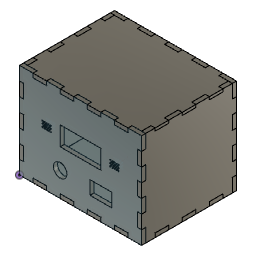
ALARMBOX (Autodesk Fusion 360 design; units mm, degrees)
Autodesk Fusion 360 part; units mm, degrees
note: some values were not read from the file. Set by a fixed rule: which sketch regions a step uses.
(part 1 of 2)
sketch "Sketch1" plane through (0, 0, 0) normal (0, 0, 1) x (1, 0, 0)
sketch "Sketch2" plane through (0, 0, 0) normal (0, 0, 1) x (1, 0, 0)
sketch "Sketch3" plane through (0, 0, 0) normal (0, 1, 0) x (1, 0, 0)
  line L0 (0, 0) -> (90, 0)
  line L1 (90, 0) -> (90, -70)
  line L2 (90, -70) -> (0, -70)
  line L3 (0, -70) -> (0, 0)
  line L4 (0, 0) -> (10, 0)
  line L5 (10, 0) -> (10, -3)
  line L6 (10, -3) -> (20, -3)
  line L7 (20, -3) -> (20, 0)
  line L8 (20, 0) -> (30, 0)
  line L9 (30, 0) -> (30, -3)
  line L10 (30, -3) -> (40, -3)
  line L11 (40, -3) -> (40, 0)
  line L12 (40, 0) -> (50, 0)
  line L13 (50, 0) -> (50, -3)
  line L14 (50, -3) -> (60, -3)
  line L15 (60, -3) -> (60, 0)
  line L16 (60, 0) -> (70, 0)
  line L17 (70, 0) -> (70, -3)
  line L18 (70, -3) -> (80, -3)
  line L19 (80, -3) -> (80, 0)
  line L20 (80, 0) -> (90, 0)
  line L21 (90, 0) -> (90, -3)
  line L22 (90, 0) -> (90, -10)
  line L23 (90, -10) -> (87, -10)
  line L24 (87, -10) -> (87, -20)
  line L25 (87, -20) -> (90, -20)
  line L26 (90, -20) -> (90, -30)
  line L27 (90, -30) -> (87, -30)
  line L28 (87, -30) -> (87, -40)
  line L29 (87, -40) -> (90, -40)
  line L30 (90, -40) -> (90, -50)
  line L31 (90, -50) -> (87, -50)
  line L32 (87, -50) -> (87, -60)
  line L33 (87, -60) -> (90, -60)
  line L34 (90, -60) -> (90, -70)
  line L35 (90, -70) -> (80, -70)
  line L36 (80, -70) -> (80, -67)
  line L37 (80, -67) -> (70, -67)
  line L38 (70, -67) -> (70, -70)
  line L39 (70, -70) -> (60, -70)
  line L40 (60, -70) -> (60, -67)
  line L41 (60, -67) -> (50, -67)
  line L42 (50, -67) -> (50, -70)
  line L43 (50, -70) -> (40, -70)
  line L44 (40, -70) -> (40, -67)
  line L45 (40, -67) -> (30, -67)
  line L46 (30, -67) -> (30, -70)
  line L47 (30, -70) -> (20, -70)
  line L48 (20, -70) -> (20, -67)
  line L49 (20, -67) -> (10, -67)
  line L50 (10, -67) -> (10, -70)
  line L51 (10, -70) -> (0, -70)
  line L52 (0, -70) -> (0, -60)
  line L53 (0, -60) -> (3, -60)
  line L54 (3, -60) -> (3, -50)
  line L55 (3, -50) -> (0, -50)
  line L56 (0, -50) -> (0, -40)
  line L57 (0, -40) -> (3, -40)
  line L58 (3, -40) -> (3, -30)
  line L59 (3, -30) -> (0, -30)
  line L60 (0, -30) -> (0, -20)
  line L61 (0, -20) -> (3, -20)
  line L62 (3, -20) -> (3, -10)
  line L63 (3, -10) -> (0, -10)
  dimension "d7" = 90
  dimension "d8" = 70
  dimension "d9" = 10
  dimension "d14" = 3
  dimension "d15" = 10
  dimension "d16" = 3
  dimension "d17" = 10
  dimension "d18" = 3
  dimension "d19" = 10
  dimension "d20" = 3
  dimension "d21" = 10
  dimension "d22" = 3
  dimension "d23" = 10
  dimension "d24" = 3
  dimension "d25" = 10
  dimension "d26" = 3
  dimension "d27" = 10
  dimension "d28" = 10
  dimension "d29" = 3
  dimension "d30" = 10
  dimension "d31" = 3
  dimension "d32" = 10
  dimension "d33" = 3
  dimension "d34" = 10
  dimension "d35" = 3
  dimension "d36" = 10
  dimension "d37" = 3
  dimension "d38" = 10
  dimension "d39" = 3
  dimension "d40" = 10
  dimension "d41" = 3
  dimension "d42" = 10
  dimension "d43" = 10
  dimension "d44" = 3
  dimension "d45" = 10
  dimension "d46" = 3
  dimension "d47" = 10
  dimension "d48" = 3
  dimension "d49" = 10
  dimension "d50" = 3
  dimension "d51" = 10
  dimension "d52" = 3
  dimension "d53" = 10
  dimension "d54" = 3
  dimension "d55" = 10
  dimension "d56" = 3
  dimension "d57" = 10
  dimension "d58" = 3
  dimension "d59" = 10
  dimension "d60" = 10
  dimension "d61" = 3
  dimension "d62" = 10
  dimension "d63" = 3
  dimension "d64" = 10
  dimension "d65" = 3
  dimension "d66" = 10
  dimension "d67" = 3
  dimension "d68" = 10
  dimension "d69" = 3
  dimension "d70" = 10
  dimension "d71" = 3
  constraint horizontal L0
  constraint vertical L1
  constraint horizontal L2
  constraint vertical L3
  constraint coincident L0.start L3.end
  constraint perpendicular L3 L4
  constraint perpendicular L0 L5
  constraint perpendicular L5 L6
  constraint coincident L0 L7.end
  constraint perpendicular L0 L7
  constraint perpendicular L7 L8
  constraint perpendicular L0 L9
  constraint perpendicular L9 L10
  constraint perpendicular L0 L11
  constraint perpendicular L11 L12
  constraint perpendicular L0 L13
  constraint perpendicular L13 L14
  constraint perpendicular L0 L15
  constraint coincident L0 L16.end
  constraint perpendicular L16 L17
  constraint perpendicular L17 L18
  constraint coincident L0 L19.end
  constraint perpendicular L0 L19
  constraint coincident L0 L1.start
  constraint perpendicular L20 L21
  constraint perpendicular L0 L22
  constraint perpendicular L22 L23
  constraint perpendicular L23 L24
  constraint perpendicular L24 L25
  constraint perpendicular L25 L26
  constraint perpendicular L1 L27
  constraint perpendicular L27 L28
  constraint perpendicular L1 L29
  constraint perpendicular L29 L30
  constraint perpendicular L30 L31
  constraint perpendicular L31 L32
  constraint perpendicular L1 L33
  constraint perpendicular L2 L34
  constraint perpendicular L34 L35
  constraint perpendicular L35 L36
  constraint perpendicular L36 L37
  constraint perpendicular L2 L38
  constraint perpendicular L38 L39
  constraint perpendicular L39 L40
  constraint perpendicular L40 L41
  constraint perpendicular L2 L42
  constraint coincident L2 L43.end
  constraint perpendicular L43 L44
  constraint perpendicular L44 L45
  constraint coincident L2 L46.end
  constraint coincident L2 L47.end
  constraint perpendicular L47 L48
  constraint perpendicular L3 L49
  constraint coincident L2 L50.end
  constraint coincident L2 L3.start
  constraint coincident L3 L52.end
  constraint perpendicular L52 L53
  constraint perpendicular L53 L54
  constraint coincident L3 L55.end
  constraint coincident L3 L56.end
  constraint perpendicular L55 L56
  constraint perpendicular L56 L57
  constraint perpendicular L55 L58
  constraint coincident L3 L59.end
  constraint coincident L3 L60.end
  constraint perpendicular L59 L60
  constraint perpendicular L60 L61
  constraint perpendicular L61 L62
  constraint coincident L3 L63.end
  measures "d7" distance of L0.start L0.end
  measures "d8" distance of L0.start L2.end
  measures "d9" distance of L0.start L4.end
  measures "d14" distance of L4.end L5.end
  measures "d15" distance of L5.end L6.end
  measures "d16" distance of L6.end L7.end
  measures "d17" distance of L7.end L8.end
  measures "d18" distance of L8.end L9.end
  measures "d19" distance of L9.end L10.end
  measures "d20" distance of L10.end L11.end
  measures "d21" distance of L11.end L12.end
  measures "d22" distance of L12.end L13.end
  measures "d23" distance of L13.end L14.end
  measures "d24" distance of L14.end L15.end
  measures "d25" distance of L15.end L16.end
  measures "d26" distance of L16.end L17.end
  measures "d27" distance of L17.end L18.end
  measures "d28" distance of L19.end L0.end
  measures "d29" distance of L0.end L21.end
  measures "d30" distance of L0.end L22.end
  measures "d31" distance of L22.end L23.end
  measures "d32" distance of L23.end L24.end
  measures "d33" distance of L24.end L25.end
  measures "d34" distance of L25.end L26.end
  measures "d35" distance of L26.end L27.end
  measures "d36" distance of L27.end L28.end
  measures "d37" distance of L28.end L29.end
  measures "d38" distance of L29.end L30.end
  measures "d39" distance of L30.end L31.end
  measures "d40" distance of L31.end L32.end
  measures "d41" distance of L32.end L33.end
  measures "d42" distance of L33.end L1.end
  measures "d43" distance of L1.end L35.end
  measures "d44" distance of L35.end L36.end
  measures "d45" distance of L36.end L37.end
  measures "d46" distance of L37.end L38.end
  measures "d47" distance of L38.end L39.end
  measures "d48" distance of L39.end L40.end
  measures "d49" distance of L40.end L41.end
  measures "d50" distance of L41.end L42.end
  measures "d51" distance of L42.end L43.end
  measures "d52" distance of L43.end L44.end
  measures "d53" distance of L44.end L45.end
  measures "d54" distance of L45.end L46.end
  measures "d55" distance of L46.end L47.end
  measures "d56" distance of L47.end L48.end
  measures "d57" distance of L48.end L49.end
  measures "d58" distance of L49.end L50.end
  measures "d59" distance of L50.end L2.end
  measures "d60" distance of L2.end L52.end
  measures "d61" distance of L52.end L53.end
  measures "d62" distance of L53.end L54.end
  measures "d63" distance of L54.end L55.end
  measures "d64" distance of L55.end L56.end
  measures "d65" distance of L56.end L57.end
  measures "d66" distance of L57.end L58.end
  measures "d67" distance of L58.end L59.end
  measures "d68" distance of L59.end L60.end
  measures "d69" distance of L60.end L61.end
  measures "d70" distance of L61.end L62.end
  measures "d71" distance of L62.end L63.end
sketch "Sketch6" plane through (0, 0, 0) normal (0, 0, 1) x (1, 0, 0)
sketch "Sketch7" plane through (0, 0, 0) normal (0, 0, 1) x (1, 0, 0)
  line L0 (0, 0) -> (90, 0)
  line L1 (90, 0) -> (90, 70)
  line L2 (90, 70) -> (0, 70)
  line L3 (0, 70) -> (0, 0)
  dimension "d72" = 90
  dimension "d73" = 70
  constraint horizontal L0
  constraint vertical L1
  constraint horizontal L2
  constraint vertical L3
  constraint coincident L0.start L3.end
  measures "d72" distance of L0.start L0.end
  measures "d73" distance of L0.start L2.end
extrude "Extrude1" add sketch "Sketch7" along normal blind 3 makes body 1
extrude "Extrude2" add sketch "Sketch3" along normal blind 3 separate body contours L0 L1 L2 L3 L4 L5 L6 L7 L8 L9 L10 L11 L12 L13 L14 L15 L16 L17 L18 L19 L20 L21 L22 L23 L24 L25 L26 L27 L28 L29 L30 L31 L32 L33 L34 L35 L36 L37 L38 L39 L40 L41 L42 L43 L44 L45 L46 L47 L48 L49 L50 L51 L52 L53 L54 L55 L56 L57 L58 L59 L60 L61 L62 L63 makes body 2
ref_plane "WorkPlane1" through (45, 35, 1.5) normal (0, 1, 0) x (-1, 0, 0)
mirror "Mirror1" about plane through (45, 35, 1.5) normal (0, 1, 0) of bodies 2 makes body 3
combine "Combine1" operation cut target body 1 tool bodies 2 3 keep tools
sketch "Sketch8" plane through (90, 0, 0) normal (1, 0, 0) x (0, 1, 0)
  line L0 (67, 0) -> (67, 3)
  line L1 (3, 3) -> (3, 0)
  line L2 (3, 0) -> (67, 0)
  line L3 (0, 0) -> (70, 0)
  line L4 (70, 0) -> (70, 70)
  line L5 (70, 70) -> (0, 70)
  line L6 (0, 70) -> (0, 0)
  line L7 (0, 0) -> (10, 0)
  line L8 (10, 0) -> (10.1015, 2.9983)
  line L9 (10.1015, 2.9983) -> (20.1008, 2.8795)
  line L10 (20.1008, 2.8795) -> (20.0677, -0.1203)
  line L11 (20.0677, -0.1203) -> (30.0671, -0.2307)
  line L12 (30.0671, -0.2307) -> (30.0154, 2.7689)
  line L13 (30.0154, 2.7689) -> (40.014, 2.941)
  line L14 (40.014, 2.941) -> (40.0159, -0.059)
  line L15 (40.0159, -0.059) -> (50.0159, -0.0525)
  line L16 (50.0159, -0.0525) -> (50.0001, 2.9475)
  line L17 (50.0001, 2.9475) -> (60, 3)
  line L18 (60, 3) -> (60, 0)
  line L19 (60, 0) -> (70, 0)
  line L20 (60, 70) -> (70, 70)
  line L21 (60, 68) -> (60, 70)
  line L22 (50, 68) -> (60, 68)
  line L23 (50, 70) -> (50, 68)
  line L24 (40, 70) -> (50, 70)
  line L25 (40, 68) -> (40, 70)
  line L26 (30, 68) -> (40, 68)
  line L27 (30, 70) -> (30, 68)
  line L28 (20, 70) -> (30, 70)
  line L29 (20, 68) -> (20, 70)
  line L30 (10, 68) -> (20, 68)
  line L31 (10, 70) -> (10, 68)
  line L32 (0, 70) -> (10, 70)
  dimension "d80" = 70
  dimension "d81" = 70
  dimension "d82" = 10
  dimension "d83" = 3
  dimension "d84" = 10
  dimension "d85" = 3
  dimension "d86" = 10
  dimension "d87" = 3
  dimension "d88" = 10
  dimension "d89" = 3
  dimension "d90" = 10
  dimension "d91" = 3
  dimension "d93" = 10
  dimension "d94" = 3
  constraint horizontal L3
  constraint vertical L4
  constraint horizontal L5
  constraint vertical L6
  constraint coincident L3.start L6.end
  constraint coincident L3 L7.end
  constraint perpendicular L10 L11
  constraint perpendicular L12 L13
  constraint perpendicular L14 L15
  constraint perpendicular L16 L17
  constraint perpendicular L3 L18
  measures "d80" distance of L3.start L3.end
  measures "d81" distance of L3.start L5.end
  measures "d82" distance of L3.start L7.end
  measures "d83" distance of L7.end L8.end
  measures "d84" distance of L8.end L9.end
  measures "d85" distance of L9.end L10.end
  measures "d86" distance of L10.end L11.end
  measures "d87" distance of L11.end L12.end
  measures "d88" distance of L12.end L13.end
  measures "d89" distance of L13.end L14.end
  measures "d90" distance of L14.end L15.end
  measures "d91" distance of L15.end L16.end
  measures "d93" distance of L16.end L17.end
  measures "d94" distance of L17.end L18.end
extrude "Extrude3" add sketch "Sketch8" against normal blind 3 separate body contours L2 L3 L4 L5 L6 L7 L8 L9 L10 L12 L13 L14 L16 L17 L18 L19 L20 L21 L22 L23 L24 L25 L26 L27 L28 L29 L30 L31 L32 makes body 4
ref_plane "WorkPlane2" through (45, 35, 1.5) normal (1, 0, 0) x (0, 1, 0)
mirror "Mirror2" about plane through (45, 35, 1.5) normal (1, 0, 0) of bodies 4 makes body 5
combine "Combine2" operation cut target body 1 tool bodies 4 5 keep tools
combine "Combine3" operation cut target body 4 tool bodies 2 3 keep tools
combine "Combine4" operation cut target body 5 tool bodies 3 2 keep tools
ref_plane "WorkPlane3" through (45, 35, 70) normal (0, 0, -1) x (-1, 0, 0)
sketch "Sketch9" plane through (45, 35, 70) normal (0, 0, -1) x (1, 0, 0)
  line L0 (-45, -35) -> (45, -35)
  line L1 (45, -35) -> (45, 35)
  line L2 (45, 35) -> (-45, 35)
  line L3 (-45, 35) -> (-45, -35)
  dimension "d102" = 90
  dimension "d103" = 70
  constraint horizontal L0
  constraint vertical L1
  constraint horizontal L2
  constraint vertical L3
  measures "d102" distance of L0.start L0.end
  measures "d103" distance of L0.start L2.end
extrude "Extrude4" add sketch "Sketch9" along normal blind 3 separate body makes body 6
combine "Combine5" operation cut target body 6 tool bodies 3 2 5 4 keep tools
sketch "Sketch10" plane through (0, 0, 0) normal (0, -1, 0) x (1, 0, 0)
  line L0 (3, 20) -> (3, 10)
  line L1 (3, 10) -> (0, 10)
  line L2 (0, 10) -> (0, 0)
  line L3 (0, 0) -> (10, 0)
  line L4 (10, 0) -> (10, 3)
  line L5 (10, 3) -> (20, 3)
  line L6 (20, 3) -> (20, 0)
  line L7 (20, 0) -> (30, 0)
  line L8 (30, 0) -> (30, 3)
  line L9 (30, 3) -> (40, 3)
  line L10 (40, 3) -> (40, 0)
  line L11 (40, 0) -> (50, 0)
  line L12 (50, 0) -> (50, 3)
  line L13 (50, 3) -> (60, 3)
  line L14 (60, 3) -> (60, 0)
  line L15 (60, 0) -> (70, 0)
  line L16 (70, 0) -> (70, 3)
  line L17 (70, 3) -> (80, 3)
  line L18 (80, 3) -> (80, 0)
  line L19 (80, 0) -> (90, 0)
  line L20 (90, 0) -> (90, 10)
  line L21 (90, 10) -> (87, 10)
  line L22 (87, 10) -> (87, 20)
  line L23 (87, 20) -> (90, 20)
  line L24 (90, 20) -> (90, 30)
  line L25 (90, 30) -> (87, 30)
  line L26 (87, 30) -> (87, 40)
  line L27 (87, 40) -> (90, 40)
  line L28 (90, 40) -> (90, 50)
  line L29 (90, 50) -> (87, 50)
  line L30 (87, 50) -> (87, 60)
  line L31 (87, 60) -> (90, 60)
  line L32 (90, 60) -> (90, 70)
  line L33 (90, 70) -> (80, 70)
  line L34 (80, 70) -> (80, 67)
  line L35 (80, 67) -> (70, 67)
  line L36 (70, 67) -> (70, 70)
  line L37 (70, 70) -> (60, 70)
  line L38 (60, 70) -> (60, 67)
  line L39 (60, 67) -> (50, 67)
  line L40 (50, 67) -> (50, 70)
  line L41 (50, 70) -> (40, 70)
  line L42 (40, 70) -> (40, 67)
  line L43 (40, 67) -> (30, 67)
  line L44 (30, 67) -> (30, 70)
  line L45 (30, 70) -> (20, 70)
  line L46 (20, 70) -> (20, 67)
  line L47 (20, 67) -> (10, 67)
  line L48 (10, 67) -> (10, 70)
  line L49 (10, 70) -> (0, 70)
  line L50 (0, 70) -> (0, 60)
  line L51 (0, 60) -> (3, 60)
  line L52 (3, 60) -> (3, 50)
  line L53 (3, 50) -> (0, 50)
  line L54 (0, 50) -> (0, 40)
  line L55 (0, 40) -> (3, 40)
  line L56 (3, 40) -> (3, 30)
  line L57 (3, 30) -> (0, 30)
  line L58 (0, 30) -> (0, 20)
  line L59 (0, 20) -> (3, 20)
sketch "Sketch11" plane through (45, 0, 35) normal (0, -1, 0) x (1, 0, 0)
  line L0 (15, 7.25) -> (-15, 7.25)
  line L1 (-15, 7.25) -> (-15, -7.25)
  line L2 (-15, -7.25) -> (15, -7.25)
  line L3 (15, -7.25) -> (15, 7.25)
  line L4 (15, 7.25) -> (-15, -7.25) construction
  line L5 (-15, 7.25) -> (15, -7.25) construction
  dimension "d110" = 30
  dimension "d111" = 14.5
  constraint horizontal L0
  constraint perpendicular L0 L1
  constraint parallel L0 L2
  constraint parallel L1 L3
  constraint coincident L4 origin
  constraint coincident L5 origin
  measures "d110" distance of L1.end L2.end
  measures "d111" distance of L0.end L1.end
sketch "Sketch19" plane through (0, 0, 0) normal (0, -1, 0) x (1, 0, 0)
  line L0 (10, 25) -> (26, 25)
  line L1 (26, 25) -> (26, 15)
  line L2 (26, 15) -> (10, 15)
  line L3 (10, 15) -> (10, 25)
  circle A0 centre (35, 20) radius 5
  circle A1 centre (70, 10) radius 1
  circle A2 centre (75, 10) radius 1
  circle A3 centre (80, 10) radius 1
  circle A4 centre (75, 15) radius 1
  circle A5 centre (80, 15) radius 1
  circle A6 centre (70, 15) radius 1
  circle A7 centre (70, 20) radius 1
  circle A8 centre (75, 20) radius 1
  circle A9 centre (80, 20) radius 1
  dimension "d140" = 16
  dimension "d141" = 2
  constraint horizontal L0
  constraint vertical L1
  constraint horizontal L2
  constraint vertical L3
  measures "d140" distance of L0.start L0.end
  measures "d141" diameter of A1
sketch "Sketch22" plane through (90, 0, 0) normal (1, 0, 0) x (0, 1, 0)
  line L0 (67, 0) -> (67, 10)
  line L1 (67, 10) -> (70, 10)
  line L2 (70, 10) -> (70, 20)
  line L3 (70, 20) -> (67, 20)
  line L4 (67, 20) -> (67, 30)
  line L5 (67, 30) -> (70, 30)
  line L6 (70, 30) -> (70, 40)
  line L7 (70, 40) -> (67, 40)
  line L8 (67, 40) -> (67, 50)
  line L9 (67, 50) -> (70, 50)
  line L10 (70, 50) -> (70, 60)
  line L11 (70, 60) -> (67, 60)
  line L12 (67, 60) -> (67, 70)
  line L13 (67, 70) -> (60, 70)
  line L14 (60, 70) -> (60, 68)
  line L15 (60, 68) -> (50, 68)
  line L16 (50, 68) -> (50, 70)
  line L17 (50, 70) -> (40, 70)
  line L18 (40, 70) -> (40, 68)
  line L19 (40, 68) -> (30, 68)
  line L20 (30, 68) -> (30, 70)
  line L21 (30, 70) -> (20, 70)
  line L22 (20, 70) -> (20, 68)
  line L23 (20, 68) -> (10, 68)
  line L24 (10, 68) -> (10, 70)
  line L25 (10, 70) -> (3, 70)
  line L26 (3, 70) -> (3, 60)
  line L27 (3, 60) -> (0, 60)
  line L28 (0, 60) -> (0, 50)
  line L29 (0, 50) -> (3, 50)
  line L30 (3, 50) -> (3, 40)
  line L31 (3, 40) -> (0, 40)
  line L32 (0, 40) -> (0, 30)
  line L33 (0, 30) -> (3, 30)
  line L34 (3, 30) -> (3, 20)
  line L35 (3, 20) -> (0, 20)
  line L36 (0, 20) -> (0, 10)
  line L37 (0, 10) -> (3, 10)
  line L38 (3, 10) -> (3, 0)
  line L39 (3, 0) -> (10, 0)
  line L40 (10, 0) -> (10.1015, 2.9983)
  line L41 (10.1015, 2.9983) -> (20.1008, 2.8795)
  line L42 (20.1008, 2.8795) -> (20.069, 0)
  line L43 (20.069, 0) -> (30.0631, 0)
  line L44 (30.0631, 0) -> (30.0154, 2.7689)
  line L45 (30.0154, 2.7689) -> (40.014, 2.941)
  line L46 (40.014, 2.941) -> (40.0159, 0)
  line L47 (40.0159, 0) -> (50.0156, 0)
  line L48 (50.0156, 0) -> (50.0001, 2.9475)
  line L49 (50.0001, 2.9475) -> (60, 3)
  line L50 (60, 3) -> (60, 0)
  line L51 (60, 0) -> (67, 0)
  spline S0 degree 3 poles (30.3334, 17.2621) (27.6065, 17.2805) (25.3535, 17.304) (25.3268, 17.3143) knots 0 0 0 0 1 1 1 1
  spline S1 degree 3 poles (25.3268, 17.3143) (25.288, 17.3293) (25.2793, 20.764) (25.2835, 34.3244) knots 0 0 0 0 1 1 1 1
  spline S2 degree 3 poles (25.2835, 34.3244) (25.2865, 43.6695) (25.3034, 52.4586) (25.3211, 53.8556) knots 0 0 0 0 1 1 1 1
  spline S3 degree 3 poles (25.3211, 53.8556) (25.3388, 55.2526) (25.3523, 56.5801) (25.351, 56.8056) knots 0 0 0 0 1 1 1 1
  line L52 (25.351, 56.8056) -> (25.3489, 57.2156)
  line L53 (25.3489, 57.2156) -> (28.7453, 57.2156)
  spline S4 degree 3 poles (28.7453, 57.2156) (30.6133, 57.2156) (34.6484, 57.2036) (37.7122, 57.189) knots 0 0 0 0 1 1 1 1
  line L54 (37.7122, 57.189) -> (43.2827, 57.1624)
  line L55 (43.2827, 57.1624) -> (43.2827, 37.189)
  line L56 (43.2827, 37.189) -> (43.2827, 17.2156)
  line L57 (43.2827, 17.2156) -> (39.2871, 17.2222)
  spline S5 degree 3 poles (39.2871, 17.2222) (37.0895, 17.2258) (33.0604, 17.2438) (30.3335, 17.2621) knots 0 0 0 0 1 1 1 1
  line L58 (30.3335, 17.2621) -> (30.3334, 17.2621)
  spline S6 degree 3 poles (33.2888, 22.5751) (41.3514, 22.6218) (42.7639, 22.6426) (42.7909, 22.7151) knots 0 0 0 0 1 1 1 1
  spline S7 degree 3 poles (42.7909, 22.7151) (42.8012, 22.7428) (42.8305, 24.2032) (42.856, 25.9605) knots 0 0 0 0 1 1 1 1
  line L59 (42.856, 25.9605) -> (42.9023, 29.1556)
  line L60 (42.9023, 29.1556) -> (42.7833, 29.4876)
  spline S8 degree 3 poles (42.7833, 29.4876) (42.5195, 30.2241) (41.9203, 31.2894) (41.3924, 31.9605) knots 0 0 0 0 1 1 1 1
  spline S9 degree 3 poles (41.3924, 31.9605) (40.7567, 32.7688) (39.6052, 33.7374) (38.5579, 34.3448) knots 0 0 0 0 1 1 1 1
  spline S10 degree 3 poles (38.5579, 34.3448) (37.5747, 34.9149) (36.5377, 35.28) (35.5053, 35.4196) knots 0 0 0 0 1 1 1 1
  spline S11 degree 3 poles (35.5053, 35.4196) (34.921, 35.4986) (33.7003, 35.4896) (33.1983, 35.4026) knots 0 0 0 0 1 1 1 1
  spline S12 degree 3 poles (33.1983, 35.4026) (31.3706, 35.086) (29.8426, 34.4023) (28.5057, 33.303) knots 0 0 0 0 1 1 1 1
  spline S13 degree 3 poles (28.5057, 33.303) (27.7205, 32.6573) (27.2357, 32.0549) (26.5364, 30.8556) knots 0 0 0 0 1 1 1 1
  spline S14 degree 3 poles (26.5364, 30.8556) (26.0363, 29.998) (25.8292, 29.5866) (25.7007, 29.1956) knots 0 0 0 0 1 1 1 1
  line L61 (25.7007, 29.1956) -> (25.6087, 28.9156)
  line L62 (25.6087, 28.9156) -> (25.6229, 25.7556)
  spline S15 degree 3 poles (25.6229, 25.7556) (25.6307, 24.0176) (25.6449, 22.5821) (25.6544, 22.5656) knots 0 0 0 0 1 1 1 1
  spline S16 degree 3 poles (25.6544, 22.5656) (25.6758, 22.5283) (25.1001, 22.5276) (33.2888, 22.5751) knots 0 0 0 0 1 1 1 1
  spline S17 degree 3 poles (42.8222, 31.3561) (42.8364, 31.4658) (42.8495, 32.6778) (42.8514, 34.0493) knots 0 0 0 0 1 1 1 1
  line L63 (42.8514, 34.0493) -> (42.8548, 36.5429)
  line L64 (42.8548, 36.5429) -> (42.0114, 37.9893)
  spline S18 degree 3 poles (42.0114, 37.9893) (40.6971, 40.2431) (37.0338, 46.4917) (36.6552, 47.1256) knots 0 0 0 0 1 1 1 1
  spline S19 degree 3 poles (36.6552, 47.1256) (36.468, 47.4391) (36.2989, 47.6956) (36.2795, 47.6956) knots 0 0 0 0 1 1 1 1
  spline S20 degree 3 poles (36.2795, 47.6956) (36.2601, 47.6956) (36.1261, 47.6342) (35.9817, 47.5592) knots 0 0 0 0 1 1 1 1
  spline S21 degree 3 poles (35.9817, 47.5592) (35.8373, 47.4841) (35.6446, 47.4002) (35.5534, 47.3727) knots 0 0 0 0 1 1 1 1
  spline S22 degree 3 poles (35.5534, 47.3727) (35.4623, 47.3452) (35.372, 47.3031) (35.3528, 47.2791) knots 0 0 0 0 1 1 1 1
  spline S23 degree 3 poles (35.3528, 47.2791) (35.331, 47.252) (35.5215, 46.5669) (35.8599, 45.4556) knots 0 0 0 0 1 1 1 1
  spline S24 degree 3 poles (35.8599, 45.4556) (36.4697, 43.4532) (36.8576, 42.1294) (37.8758, 38.5756) knots 0 0 0 0 1 1 1 1
  spline S25 degree 3 poles (37.8758, 38.5756) (38.5788, 36.1222) (38.8741, 35.1608) (39.0062, 34.8956) knots 0 0 0 0 1 1 1 1
  spline S26 degree 3 poles (39.0062, 34.8956) (39.1457, 34.6156) (39.4722, 34.1806) (39.6545, 34.0319) knots 0 0 0 0 1 1 1 1
  spline S27 degree 3 poles (39.6545, 34.0319) (40.6796, 33.1956) (40.9885, 32.8997) (41.487, 32.277) knots 0 0 0 0 1 1 1 1
  spline S28 degree 3 poles (41.487, 32.277) (41.7153, 31.9917) (41.9661, 31.6855) (42.0443, 31.5965) knots 0 0 0 0 1 1 1 1
  spline S29 degree 3 poles (42.0443, 31.5965) (42.2019, 31.4172) (42.647, 31.1277) (42.7381, 31.1453) knots 0 0 0 0 1 1 1 1
  spline S30 degree 3 poles (42.7381, 31.1453) (42.7763, 31.1526) (42.8054, 31.2255) (42.8222, 31.3561) knots 0 0 0 0 1 1 1 1
  spline S31 degree 3 poles (26.0309, 31.2969) (26.3536, 31.4211) (26.5173, 31.5657) (26.921, 32.083) knots 0 0 0 0 1 1 1 1
  spline S32 degree 3 poles (26.921, 32.083) (27.4185, 32.7205) (28.0737, 33.3594) (28.6637, 33.7822) knots 0 0 0 0 1 1 1 1
  spline S33 degree 3 poles (28.6637, 33.7822) (28.9297, 33.9728) (29.1939, 34.1798) (29.2507, 34.2422) knots 0 0 0 0 1 1 1 1
  spline S34 degree 3 poles (29.2507, 34.2422) (29.4833, 34.4975) (29.598, 34.7916) (30.0408, 36.2669) knots 0 0 0 0 1 1 1 1
  spline S35 degree 3 poles (30.0408, 36.2669) (30.2866, 37.0857) (30.909, 39.0426) (31.424, 40.6156) knots 0 0 0 0 1 1 1 1
  spline S36 degree 3 poles (31.424, 40.6156) (31.939, 42.1886) (32.5088, 43.9706) (32.6903, 44.5756) knots 0 0 0 0 1 1 1 1
  spline S37 degree 3 poles (32.6903, 44.5756) (32.8719, 45.1806) (33.1347, 46.0335) (33.2744, 46.4709) knots 0 0 0 0 1 1 1 1
  spline S38 degree 3 poles (33.2744, 46.4709) (33.4853, 47.1311) (33.5196, 47.2751) (33.4766, 47.3182) knots 0 0 0 0 1 1 1 1
  spline S39 degree 3 poles (33.4766, 47.3182) (33.4482, 47.3468) (33.2411, 47.451) (33.0166, 47.5499) knots 0 0 0 0 1 1 1 1
  spline S40 degree 3 poles (33.0166, 47.5499) (32.6354, 47.7177) (32.604, 47.7252) (32.5447, 47.6626) knots 0 0 0 0 1 1 1 1
  spline S41 degree 3 poles (32.5447, 47.6626) (32.5098, 47.6258) (31.9776, 46.7496) (31.3621, 45.7156) knots 0 0 0 0 1 1 1 1
  spline S42 degree 3 poles (31.3621, 45.7156) (29.4896, 42.5702) (27.0499, 38.4924) (26.0731, 36.8756) knots 0 0 0 0 1 1 1 1
  line L65 (26.0731, 36.8756) -> (25.6865, 36.2356)
  line L66 (25.6865, 36.2356) -> (25.6657, 33.7756)
  spline S43 degree 3 poles (25.6657, 33.7756) (25.6542, 32.4226) (25.6517, 31.2931) (25.6601, 31.2656) knots 0 0 0 0 1 1 1 1
  spline S44 degree 3 poles (25.6601, 31.2656) (25.6818, 31.1945) (25.7881, 31.2035) (26.0309, 31.2969) knots 0 0 0 0 1 1 1 1
  spline S45 degree 3 poles (30.8329, 35.052) (31.6951, 35.4257) (32.7366, 35.6956) (33.3163, 35.6956) knots 0 0 0 0 1 1 1 1
  spline S46 degree 3 poles (33.3163, 35.6956) (33.6245, 35.6956) (33.7747, 35.7589) (33.9553, 35.9647) knots 0 0 0 0 1 1 1 1
  line L67 (33.9553, 35.9647) -> (34.0968, 36.1261)
  line L68 (34.0968, 36.1261) -> (34.1203, 36.7009)
  spline S47 degree 3 poles (34.1203, 36.7009) (34.1332, 37.017) (34.1482, 39.5076) (34.1537, 42.2356) knots 0 0 0 0 1 1 1 1
  line L69 (34.1537, 42.2356) -> (34.1637, 47.1956)
  line L70 (34.1637, 47.1956) -> (34.0373, 47.2081)
  spline S48 degree 3 poles (34.0373, 47.2081) (33.9296, 47.2188) (33.9048, 47.2042) (33.8696, 47.109) knots 0 0 0 0 1 1 1 1
  spline S49 degree 3 poles (33.8696, 47.109) (33.8263, 46.9917) (32.6937, 43.3148) (31.9865, 40.9956) knots 0 0 0 0 1 1 1 1
  spline S50 degree 3 poles (31.9865, 40.9956) (31.7584, 40.2476) (31.2669, 38.6538) (30.8943, 37.4539) knots 0 0 0 0 1 1 1 1
  spline S51 degree 3 poles (30.8943, 37.4539) (30.5216, 36.2539) (30.2167, 35.2067) (30.2167, 35.1267) knots 0 0 0 0 1 1 1 1
  spline S52 degree 3 poles (30.2167, 35.1267) (30.2167, 35.0018) (30.2936, 34.8556) (30.3594, 34.8556) knots 0 0 0 0 1 1 1 1
  spline S53 degree 3 poles (30.3594, 34.8556) (30.3706, 34.8556) (30.5837, 34.944) (30.8329, 35.052) knots 0 0 0 0 1 1 1 1
  spline S54 degree 3 poles (38.3815, 34.973) (38.4463, 35.0976) (38.4305, 35.201) (38.268, 35.7146) knots 0 0 0 0 1 1 1 1
  spline S55 degree 3 poles (38.268, 35.7146) (38.1196, 36.1839) (37.7415, 37.5168) (36.3216, 42.5756) knots 0 0 0 0 1 1 1 1
  spline S56 degree 3 poles (36.3216, 42.5756) (35.4602, 45.6445) (35.297, 46.2195) (35.1326, 46.7656) knots 0 0 0 0 1 1 1 1
  line L71 (35.1326, 46.7656) -> (34.9971, 47.2156)
  line L72 (34.9971, 47.2156) -> (34.7457, 47.2156)
  spline S57 degree 3 poles (34.7457, 47.2156) (34.5722, 47.2156) (34.4932, 47.2001) (34.4908, 47.1656) knots 0 0 0 0 1 1 1 1
  spline S58 degree 3 poles (34.4908, 47.1656) (34.4778, 46.9728) (34.4992, 40.6508) (34.5197, 38.639) knots 0 0 0 0 1 1 1 1
  line L73 (34.5197, 38.639) -> (34.545, 36.1624)
  line L74 (34.545, 36.1624) -> (34.6815, 36.0069)
  spline S59 degree 3 poles (34.6815, 36.0069) (34.7566, 35.9214) (34.8546, 35.8313) (34.8992, 35.8066) knots 0 0 0 0 1 1 1 1
  spline S60 degree 3 poles (34.8992, 35.8066) (34.9438, 35.782) (35.2341, 35.7289) (35.5442, 35.6885) knots 0 0 0 0 1 1 1 1
  spline S61 degree 3 poles (35.5442, 35.6885) (36.226, 35.5999) (37.0666, 35.3717) (37.7041, 35.1022) knots 0 0 0 0 1 1 1 1
  spline S62 degree 3 poles (37.7041, 35.1022) (38.2287, 34.8805) (38.3239, 34.8623) (38.3815, 34.973) knots 0 0 0 0 1 1 1 1
  spline S63 degree 3 poles (42.8081, 39.0236) (42.8434, 39.0599) (42.8548, 39.6648) (42.8548, 41.5012) knots 0 0 0 0 1 1 1 1
  line L75 (42.8548, 41.5012) -> (42.8548, 43.9307)
  line L76 (42.8548, 43.9307) -> (42.695, 44.1232)
  spline S64 degree 3 poles (42.695, 44.1232) (42.1455, 44.7851) (41.8818, 45.0114) (40.6383, 45.8881) knots 0 0 0 0 1 1 1 1
  spline S65 degree 3 poles (40.6383, 45.8881) (39.9646, 46.363) (38.9044, 47.1142) (38.2823, 47.5572) knots 0 0 0 0 1 1 1 1
  spline S66 degree 3 poles (38.2823, 47.5572) (37.6601, 48.0003) (37.1291, 48.3769) (37.1021, 48.394) knots 0 0 0 0 1 1 1 1
  spline S67 degree 3 poles (37.1021, 48.394) (37.0494, 48.4276) (36.633, 48.0355) (36.633, 47.9523) knots 0 0 0 0 1 1 1 1
  spline S68 degree 3 poles (36.633, 47.9523) (36.633, 47.9128) (37.6617, 46.1622) (40.3567, 41.6156) knots 0 0 0 0 1 1 1 1
  spline S69 degree 3 poles (40.3567, 41.6156) (41.5801, 39.5517) (41.7611, 39.2653) (41.8959, 39.1796) knots 0 0 0 0 1 1 1 1
  spline S70 degree 3 poles (41.8959, 39.1796) (42.1555, 39.0145) (42.7075, 38.9201) (42.8081, 39.0236) knots 0 0 0 0 1 1 1 1
  spline S71 degree 3 poles (26.7408, 39.194) (27.0325, 39.3422) (27.0391, 39.3491) (27.3172, 39.7898) knots 0 0 0 0 1 1 1 1
  spline S72 degree 3 poles (27.3172, 39.7898) (27.4719, 40.035) (28.4267, 41.6306) (29.439, 43.3356) knots 0 0 0 0 1 1 1 1
  spline S73 degree 3 poles (29.439, 43.3356) (30.4513, 45.0406) (31.4866, 46.7822) (31.7397, 47.2059) knots 0 0 0 0 1 1 1 1
  spline S74 degree 3 poles (31.7397, 47.2059) (31.9928, 47.6295) (32.1999, 47.9902) (32.1999, 48.0074) knots 0 0 0 0 1 1 1 1
  spline S75 degree 3 poles (32.1999, 48.0074) (32.1999, 48.0246) (32.1145, 48.1252) (32.01, 48.231) knots 0 0 0 0 1 1 1 1
  spline S76 degree 3 poles (32.01, 48.231) (31.8348, 48.4085) (31.813, 48.4195) (31.7281, 48.373) knots 0 0 0 0 1 1 1 1
  spline S77 degree 3 poles (31.7281, 48.373) (31.6142, 48.3107) (28.1451, 45.9343) (27.2419, 45.2999) knots 0 0 0 0 1 1 1 1
  spline S78 degree 3 poles (27.2419, 45.2999) (26.5014, 44.7798) (26.1506, 44.4447) (25.8896, 44.0081) knots 0 0 0 0 1 1 1 1
  line L77 (25.8896, 44.0081) -> (25.7147, 43.7156)
  line L78 (25.7147, 43.7156) -> (25.6896, 41.5756)
  spline S79 degree 3 poles (25.6896, 41.5756) (25.6661, 39.5716) (25.6689, 39.4267) (25.7338, 39.2956) knots 0 0 0 0 1 1 1 1
  spline S80 degree 3 poles (25.7338, 39.2956) (25.8911, 38.9779) (26.2455, 38.9421) (26.7408, 39.194) knots 0 0 0 0 1 1 1 1
  line L79 (42.7932, 45.7097) -> (42.8937, 45.7775)
  line L80 (42.8937, 45.7775) -> (42.8937, 47.3319)
  line L81 (42.8937, 47.3319) -> (42.8937, 48.8863)
  line L82 (42.8937, 48.8863) -> (42.7394, 49.0297)
  spline S81 degree 3 poles (42.7394, 49.0297) (42.6545, 49.1086) (42.4926, 49.2352) (42.3797, 49.3111) knots 0 0 0 0 1 1 1 1
  spline S82 degree 3 poles (42.3797, 49.3111) (42.1783, 49.4463) (42.1355, 49.4559) (40.2105, 49.7968) knots 0 0 0 0 1 1 1 1
  spline S83 degree 3 poles (40.2105, 49.7968) (39.1305, 49.9881) (38.1616, 50.1471) (38.0575, 50.1501) knots 0 0 0 0 1 1 1 1
  line L83 (38.0575, 50.1501) -> (37.8683, 50.1556)
  line L84 (37.8683, 50.1556) -> (37.7411, 49.7444)
  spline S84 degree 3 poles (37.7411, 49.7444) (37.6711, 49.5182) (37.5421, 49.2057) (37.4544, 49.0499) knots 0 0 0 0 1 1 1 1
  spline S85 degree 3 poles (37.4544, 49.0499) (37.3667, 48.894) (37.3059, 48.7482) (37.3194, 48.7258) knots 0 0 0 0 1 1 1 1
  spline S86 degree 3 poles (37.3194, 48.7258) (37.34, 48.6916) (40.5958, 46.4588) (41.4284, 45.908) knots 0 0 0 0 1 1 1 1
  spline S87 degree 3 poles (41.4284, 45.908) (41.5743, 45.8115) (41.7843, 45.7064) (41.8951, 45.6744) knots 0 0 0 0 1 1 1 1
  spline S88 degree 3 poles (41.8951, 45.6744) (42.1597, 45.5979) (42.6563, 45.6175) (42.7932, 45.7097) knots 0 0 0 0 1 1 1 1
  spline S89 degree 3 poles (27.2079, 45.8294) (27.3122, 45.8845) (27.9924, 46.3436) (28.7196, 46.8497) knots 0 0 0 0 1 1 1 1
  spline S90 degree 3 poles (28.7196, 46.8497) (29.4468, 47.3557) (30.3439, 47.9797) (30.7132, 48.2362) knots 0 0 0 0 1 1 1 1
  spline S91 degree 3 poles (30.7132, 48.2362) (31.0825, 48.4928) (31.4092, 48.728) (31.4393, 48.7589) knots 0 0 0 0 1 1 1 1
  spline S92 degree 3 poles (31.4393, 48.7589) (31.4862, 48.8071) (31.4639, 48.8758) (31.2817, 49.2453) knots 0 0 0 0 1 1 1 1
  spline S93 degree 3 poles (31.2817, 49.2453) (31.165, 49.482) (31.0414, 49.7971) (31.007, 49.9456) knots 0 0 0 0 1 1 1 1
  spline S94 degree 3 poles (31.007, 49.9456) (30.9518, 50.1836) (30.9336, 50.2156) (30.8535, 50.2156) knots 0 0 0 0 1 1 1 1
  spline S95 degree 3 poles (30.8535, 50.2156) (30.7483, 50.2156) (27.8067, 49.7712) (27.1474, 49.6557) knots 0 0 0 0 1 1 1 1
  spline S96 degree 3 poles (27.1474, 49.6557) (26.5905, 49.5581) (26.3602, 49.4426) (25.9886, 49.0748) knots 0 0 0 0 1 1 1 1
  line L85 (25.9886, 49.0748) -> (25.7049, 48.794)
  line L86 (25.7049, 48.794) -> (25.7151, 47.3948)
  line L87 (25.7151, 47.3948) -> (25.7254, 45.9956)
  line L88 (25.7254, 45.9956) -> (25.9755, 45.8596)
  spline S97 degree 3 poles (25.9755, 45.8596) (26.3809, 45.6391) (26.8272, 45.6282) (27.2079, 45.8294) knots 0 0 0 0 1 1 1 1
  spline S98 degree 3 poles (35.263, 47.5559) (35.7346, 47.6703) (36.1958, 47.9685) (36.6383, 48.4452) knots 0 0 0 0 1 1 1 1
  spline S99 degree 3 poles (36.6383, 48.4452) (37.0899, 48.9319) (37.4148, 49.5054) (37.5505, 50.0554) knots 0 0 0 0 1 1 1 1
  spline S100 degree 3 poles (37.5505, 50.0554) (37.6466, 50.4452) (37.6093, 51.2646) (37.4713, 51.7956) knots 0 0 0 0 1 1 1 1
  spline S101 degree 3 poles (37.4713, 51.7956) (37.3268, 52.3515) (37.1584, 52.6441) (36.7342, 53.0763) knots 0 0 0 0 1 1 1 1
  spline S102 degree 3 poles (36.7342, 53.0763) (36.1201, 53.702) (35.5016, 54.0102) (34.6068, 54.1362) knots 0 0 0 0 1 1 1 1
  spline S103 degree 3 poles (34.6068, 54.1362) (33.7711, 54.2539) (32.7766, 53.824) (32.0447, 53.0287) knots 0 0 0 0 1 1 1 1
  spline S104 degree 3 poles (32.0447, 53.0287) (31.7828, 52.7441) (31.6955, 52.6127) (31.5213, 52.2414) knots 0 0 0 0 1 1 1 1
  spline S105 degree 3 poles (31.5213, 52.2414) (31.4064, 51.9962) (31.2901, 51.6966) (31.263, 51.5756) knots 0 0 0 0 1 1 1 1
  spline S106 degree 3 poles (31.263, 51.5756) (31.1943, 51.2695) (31.2026, 50.4951) (31.278, 50.1756) knots 0 0 0 0 1 1 1 1
  spline S107 degree 3 poles (31.278, 50.1756) (31.6149, 48.7471) (32.6679, 47.7107) (33.9573, 47.5385) knots 0 0 0 0 1 1 1 1
  spline S108 degree 3 poles (33.9573, 47.5385) (34.3672, 47.4838) (35.0004, 47.4922) (35.263, 47.5559) knots 0 0 0 0 1 1 1 1
  spline S109 degree 3 poles (42.3764, 50.1384) (42.5089, 50.1837) (42.6752, 50.2608) (42.7458, 50.3098) knots 0 0 0 0 1 1 1 1
  line L89 (42.7458, 50.3098) -> (42.8742, 50.3988)
  line L90 (42.8742, 50.3988) -> (42.8742, 51.397)
  line L91 (42.8742, 51.397) -> (42.8742, 52.3952)
  line L92 (42.8742, 52.3952) -> (42.6448, 52.4888)
  spline S110 degree 3 poles (42.6448, 52.4888) (42.485, 52.554) (42.2724, 52.5948) (41.9448, 52.6231) knots 0 0 0 0 1 1 1 1
  line L93 (41.9448, 52.6231) -> (41.4743, 52.6636)
  line L94 (41.4743, 52.6636) -> (39.7828, 52.2984)
  spline S111 degree 3 poles (39.7828, 52.2984) (37.5924, 51.8255) (37.7868, 51.8843) (37.8129, 51.703) knots 0 0 0 0 1 1 1 1
  spline S112 degree 3 poles (37.8129, 51.703) (37.8246, 51.6219) (37.8544, 51.3486) (37.8792, 51.0956) knots 0 0 0 0 1 1 1 1
  spline S113 degree 3 poles (37.8792, 51.0956) (37.9039, 50.8426) (37.9309, 50.6283) (37.9392, 50.6194) knots 0 0 0 0 1 1 1 1
  spline S114 degree 3 poles (37.9392, 50.6194) (37.9474, 50.6105) (38.79, 50.4717) (39.8115, 50.311) knots 0 0 0 0 1 1 1 1
  spline S115 degree 3 poles (39.8115, 50.311) (41.8101, 49.9965) (41.9361, 49.988) (42.3764, 50.1384) knots 0 0 0 0 1 1 1 1
  spline S116 degree 3 poles (28.819, 50.3539) (29.9003, 50.496) (30.8134, 50.6234) (30.8481, 50.6371) knots 0 0 0 0 1 1 1 1
  spline S117 degree 3 poles (30.8481, 50.6371) (30.8937, 50.6551) (30.9179, 50.7357) (30.9356, 50.9288) knots 0 0 0 0 1 1 1 1
  spline S118 degree 3 poles (30.9356, 50.9288) (30.949, 51.0755) (30.979, 51.3271) (31.0023, 51.4878) knots 0 0 0 0 1 1 1 1
  spline S119 degree 3 poles (31.0023, 51.4878) (31.028, 51.6648) (31.0307, 51.7944) (31.0091, 51.8166) knots 0 0 0 0 1 1 1 1
  spline S120 degree 3 poles (31.0091, 51.8166) (30.9687, 51.8581) (27.7097, 52.5973) (27.332, 52.6507) knots 0 0 0 0 1 1 1 1
  spline S121 degree 3 poles (27.332, 52.6507) (26.9138, 52.7097) (26.3779, 52.6072) (25.9392, 52.3843) knots 0 0 0 0 1 1 1 1
  line L95 (25.9392, 52.3843) -> (25.7254, 52.2756)
  line L96 (25.7254, 52.2756) -> (25.7148, 51.5257)
  line L97 (25.7148, 51.5257) -> (25.7042, 50.7757)
  line L98 (25.7042, 50.7757) -> (25.8605, 50.6013)
  spline S122 degree 3 poles (25.8605, 50.6013) (26.0767, 50.3601) (26.5129, 50.1306) (26.8142, 50.0996) knots 0 0 0 0 1 1 1 1
  spline S123 degree 3 poles (26.8142, 50.0996) (26.8356, 50.0974) (27.7377, 50.2119) (28.819, 50.3539) knots 0 0 0 0 1 1 1 1
  spline S124 degree 3 poles (31.2891, 52.4056) (31.4403, 52.6725) (31.6707, 52.9913) (31.9349, 53.2991) knots 0 0 0 0 1 1 1 1
  spline S125 degree 3 poles (31.9349, 53.2991) (32.0593, 53.444) (32.1609, 53.579) (32.1607, 53.5991) knots 0 0 0 0 1 1 1 1
  spline S126 degree 3 poles (32.1607, 53.5991) (32.1605, 53.6192) (31.9112, 53.7665) (31.6066, 53.9264) knots 0 0 0 0 1 1 1 1
  line L99 (31.6066, 53.9264) -> (31.0528, 54.2172)
  line L100 (31.0528, 54.2172) -> (29.0233, 54.2164)
  spline S127 degree 3 poles (29.0233, 54.2164) (27.874, 54.216) (26.9844, 54.2001) (26.9723, 54.1799) knots 0 0 0 0 1 1 1 1
  spline S128 degree 3 poles (26.9723, 54.1799) (26.9401, 54.1264) (27.0547, 53.8694) (27.2473, 53.563) knots 0 0 0 0 1 1 1 1
  spline S129 degree 3 poles (27.2473, 53.563) (27.382, 53.3487) (27.4553, 53.2737) (27.5896, 53.2126) knots 0 0 0 0 1 1 1 1
  spline S130 degree 3 poles (27.5896, 53.2126) (27.7823, 53.1249) (30.9679, 52.2218) (31.0977, 52.218) knots 0 0 0 0 1 1 1 1
  spline S131 degree 3 poles (31.0977, 52.218) (31.1578, 52.2163) (31.2119, 52.2693) (31.2891, 52.4056) knots 0 0 0 0 1 1 1 1
  spline S132 degree 3 poles (39.2713, 52.5945) (40.8579, 52.9616) (41.1054, 53.0499) (41.4671, 53.3775) knots 0 0 0 0 1 1 1 1
  spline S133 degree 3 poles (41.4671, 53.3775) (41.6705, 53.5616) (41.8716, 53.8686) (41.9065, 54.0484) knots 0 0 0 0 1 1 1 1
  line L101 (41.9065, 54.0484) -> (41.9313, 54.1756)
  line L102 (41.9313, 54.1756) -> (39.8363, 54.1729)
  line L103 (39.8363, 54.1729) -> (37.7413, 54.1701)
  line L104 (37.7413, 54.1701) -> (37.2383, 53.8829)
  spline S134 degree 3 poles (37.2383, 53.8829) (36.9617, 53.7249) (36.7293, 53.5759) (36.7218, 53.5518) knots 0 0 0 0 1 1 1 1
  spline S135 degree 3 poles (36.7218, 53.5518) (36.7144, 53.5277) (36.849, 53.3477) (37.0209, 53.1518) knots 0 0 0 0 1 1 1 1
  spline S136 degree 3 poles (37.0209, 53.1518) (37.1928, 52.9559) (37.3956, 52.6741) (37.4715, 52.5256) knots 0 0 0 0 1 1 1 1
  spline S137 degree 3 poles (37.4715, 52.5256) (37.5866, 52.3003) (37.6258, 52.2556) (37.7083, 52.2556) knots 0 0 0 0 1 1 1 1
  spline S138 degree 3 poles (37.7083, 52.2556) (37.7626, 52.2556) (38.466, 52.4081) (39.2713, 52.5945) knots 0 0 0 0 1 1 1 1
  spline S139 degree 3 poles (32.9091, 54.004) (33.0965, 54.0856) (33.2499, 54.1666) (33.2499, 54.184) knots 0 0 0 0 1 1 1 1
  spline S140 degree 3 poles (33.2499, 54.184) (33.2499, 54.2014) (32.9611, 54.2156) (32.6082, 54.2156) knots 0 0 0 0 1 1 1 1
  spline S141 degree 3 poles (32.6082, 54.2156) (32.2124, 54.2156) (31.9666, 54.2005) (31.9666, 54.1762) knots 0 0 0 0 1 1 1 1
  spline S142 degree 3 poles (31.9666, 54.1762) (31.9666, 54.1374) (32.4547, 53.8614) (32.53, 53.8576) knots 0 0 0 0 1 1 1 1
  spline S143 degree 3 poles (32.53, 53.8576) (32.5511, 53.8565) (32.7217, 53.9224) (32.9091, 54.004) knots 0 0 0 0 1 1 1 1
  line L105 (36.5659, 54.0056) -> (36.8469, 54.1556)
  line L106 (36.8469, 54.1556) -> (36.5455, 54.1673)
  spline S144 degree 3 poles (36.5455, 54.1673) (36.3797, 54.1737) (36.1085, 54.1737) (35.9428, 54.1673) knots 0 0 0 0 1 1 1 1
  line L107 (35.9428, 54.1673) -> (35.6414, 54.1556)
  line L108 (35.6414, 54.1556) -> (35.933, 54.0088)
  spline S145 degree 3 poles (35.933, 54.0088) (36.0934, 53.928) (36.2382, 53.8605) (36.2548, 53.8588) knots 0 0 0 0 1 1 1 1
  spline S146 degree 3 poles (36.2548, 53.8588) (36.2714, 53.857) (36.4114, 53.9231) (36.5659, 54.0056) knots 0 0 0 0 1 1 1 1
sketch "Sketch23" plane through (0, 3, 0) normal (0, 1, 0) x (-1, 0, 0)
  line L0 (-3, 10) -> (-3, 20)
  line L1 (-3, 20) -> (0, 20)
  line L2 (0, 20) -> (0, 30)
  line L3 (0, 30) -> (-3, 30)
  line L4 (-3, 30) -> (-3, 40)
  line L5 (-3, 40) -> (0, 40)
  line L6 (0, 40) -> (0, 50)
  line L7 (0, 50) -> (-3, 50)
  line L8 (-3, 50) -> (-3, 60)
  line L9 (-3, 60) -> (0, 60)
  line L10 (0, 60) -> (0, 70)
  line L11 (0, 70) -> (-10, 70)
  line L12 (-10, 70) -> (-10, 67)
  line L13 (-10, 67) -> (-20, 67)
  line L14 (-20, 67) -> (-20, 70)
  line L15 (-20, 70) -> (-30, 70)
  line L16 (-30, 70) -> (-30, 67)
  line L17 (-30, 67) -> (-40, 67)
  line L18 (-40, 67) -> (-40, 70)
  line L19 (-40, 70) -> (-50, 70)
  line L20 (-50, 70) -> (-50, 67)
  line L21 (-50, 67) -> (-60, 67)
  line L22 (-60, 67) -> (-60, 70)
  line L23 (-60, 70) -> (-70, 70)
  line L24 (-70, 70) -> (-70, 67)
  line L25 (-70, 67) -> (-80, 67)
  line L26 (-80, 67) -> (-80, 70)
  line L27 (-80, 70) -> (-90, 70)
  line L28 (-90, 70) -> (-90, 60)
  line L29 (-90, 60) -> (-87, 60)
  line L30 (-87, 60) -> (-87, 50)
  line L31 (-87, 50) -> (-90, 50)
  line L32 (-90, 50) -> (-90, 40)
  line L33 (-90, 40) -> (-87, 40)
  line L34 (-87, 40) -> (-87, 30)
  line L35 (-87, 30) -> (-90, 30)
  line L36 (-90, 30) -> (-90, 20)
  line L37 (-90, 20) -> (-87, 20)
  line L38 (-87, 20) -> (-87, 10)
  line L39 (-87, 10) -> (-90, 10)
  line L40 (-90, 10) -> (-90, 0)
  line L41 (-90, 0) -> (-80, 0)
  line L42 (-80, 0) -> (-80, 3)
  line L43 (-80, 3) -> (-70, 3)
  line L44 (-70, 3) -> (-70, 0)
  line L45 (-70, 0) -> (-60, 0)
  line L46 (-60, 0) -> (-60, 3)
  line L47 (-60, 3) -> (-50, 3)
  line L48 (-50, 3) -> (-50, 0)
  line L49 (-50, 0) -> (-40, 0)
  line L50 (-40, 0) -> (-40, 3)
  line L51 (-40, 3) -> (-30, 3)
  line L52 (-30, 3) -> (-30, 0)
  line L53 (-30, 0) -> (-20, 0)
  line L54 (-20, 0) -> (-20, 3)
  line L55 (-20, 3) -> (-10, 3)
  line L56 (-10, 3) -> (-10, 0)
  line L57 (-10, 0) -> (0, 0)
  line L58 (0, 0) -> (0, 10)
  line L59 (0, 10) -> (-3, 10)
  circle A0 centre (-61, 43.25) radius 0.5
  circle A1 centre (-61, 26.75) radius 0.5
  circle A2 centre (-29, 43.25) radius 0.5
  circle A3 centre (-29, 26.75) radius 0.5
  dimension "d148" = 1
  dimension "d151" = 1
  dimension "d154" = 1
  dimension "d157" = 1
  measures "d148" diameter of A0
  measures "d151" diameter of A1
  measures "d154" diameter of A2
  measures "d157" diameter of A3
sketch "Sketch31" plane through (0, 0, 0) normal (0, -1, 0) x (1, 0, 0)
  line L0 (3, 20) -> (3, 10)
  line L1 (3, 10) -> (0, 10)
  line L2 (0, 10) -> (0, 0)
  line L3 (0, 0) -> (10, 0)
  line L4 (10, 0) -> (10, 3)
  line L5 (10, 3) -> (20, 3)
  line L6 (20, 3) -> (20, 0)
  line L7 (20, 0) -> (30, 0)
  line L8 (30, 0) -> (30, 3)
  line L9 (30, 3) -> (40, 3)
  line L10 (40, 3) -> (40, 0)
  line L11 (40, 0) -> (50, 0)
  line L12 (50, 0) -> (50, 3)
  line L13 (50, 3) -> (60, 3)
  line L14 (60, 3) -> (60, 0)
  line L15 (60, 0) -> (70, 0)
  line L16 (70, 0) -> (70, 3)
  line L17 (70, 3) -> (80, 3)
  line L18 (80, 3) -> (80, 0)
  line L19 (80, 0) -> (90, 0)
  line L20 (90, 0) -> (90, 10)
  line L21 (90, 10) -> (87, 10)
  line L22 (87, 10) -> (87, 20)
  line L23 (87, 20) -> (90, 20)
  line L24 (90, 20) -> (90, 30)
  line L25 (90, 30) -> (87, 30)
  line L26 (87, 30) -> (87, 40)
  line L27 (87, 40) -> (90, 40)
  line L28 (90, 40) -> (90, 50)
  line L29 (90, 50) -> (87, 50)
  line L30 (87, 50) -> (87, 60)
  line L31 (87, 60) -> (90, 60)
  line L32 (90, 60) -> (90, 70)
  line L33 (90, 70) -> (80, 70)
  line L34 (80, 70) -> (80, 67)
  line L35 (80, 67) -> (70, 67)
  line L36 (70, 67) -> (70, 70)
  line L37 (70, 70) -> (60, 70)
  line L38 (60, 70) -> (60, 67)
  line L39 (60, 67) -> (50, 67)
  line L40 (50, 67) -> (50, 70)
  line L41 (50, 70) -> (40, 70)
  line L42 (40, 70) -> (40, 67)
  line L43 (40, 67) -> (30, 67)
  line L44 (30, 67) -> (30, 70)
  line L45 (30, 70) -> (20, 70)
  line L46 (20, 70) -> (20, 67)
  line L47 (20, 67) -> (10, 67)
  line L48 (10, 67) -> (10, 70)
  line L49 (10, 70) -> (0, 70)
  line L50 (0, 70) -> (0, 60)
  line L51 (0, 60) -> (3, 60)
  line L52 (3, 60) -> (3, 50)
  line L53 (3, 50) -> (0, 50)
  line L54 (0, 50) -> (0, 40)
  line L55 (0, 40) -> (3, 40)
  line L56 (3, 40) -> (3, 30)
  line L57 (3, 30) -> (0, 30)
  line L58 (0, 30) -> (0, 20)
  line L59 (0, 20) -> (3, 20)
  line L60 (60, 47) -> (30, 47)
  line L61 (30, 47) -> (30, 33)
  line L62 (30, 33) -> (60, 33)
  line L63 (60, 33) -> (60, 47)
  line L64 (60, 47) -> (30, 33) construction
  line L65 (30, 47) -> (60, 33) construction
  circle A0 centre (30, 18) radius 5
  line L66 (68, 23) -> (52, 23)
  line L67 (52, 23) -> (52, 13)
  line L68 (52, 13) -> (68, 13)
  line L69 (68, 13) -> (68, 23)
  line L70 (68, 23) -> (52, 13) construction
  line L71 (52, 23) -> (68, 13) construction
  point P0 (45, 40)
  point P1 (60, 18)
  dimension "d162" = 45
  dimension "d163" = 30
  dimension "d164" = 14
  dimension "d165" = 10
  dimension "d166" = 16
  dimension "d167" = 10
  constraint horizontal L60
  constraint perpendicular L60 L61
  constraint parallel L60 L62
  constraint parallel L61 L63
  constraint coincident L64 P0
  constraint coincident L65 P0
  constraint horizontal L66
  constraint perpendicular L66 L67
  constraint parallel L66 L68
  constraint parallel L67 L69
  constraint coincident L70 P1
  constraint coincident L71 P1
  measures "d162" distance of L54.end P0
  measures "d163" distance of L61.end L62.end
  measures "d164" distance of L60.end L61.end
  measures "d165" diameter of A0
  measures "d166" distance of L67.end L68.end
  measures "d167" distance of L66.end L67.end
extrude "Extrude14" cut sketch "Sketch31" against normal blind 3 contours L60 L61 L62 L63 | A0 | L66 L67 L68 L69 bodies 2